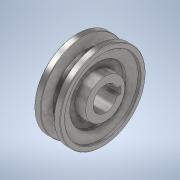
# Autodesk Inventor part: Pulley
Saved by Autodesk Inventor 2021 (Build 250183000, 183)
## iProperties
Created: 2021-07-07
Part Number: Pulley
Material: Steel, Cast
Document SubType Name: Modeling
Designer: MOGIRE
Density: 7.85 g/cm^3
Appearance: Semi-Polished
Author: MOGIRE
Autodesk Inventor part; units mm, degrees
ref_plane "YZ Plane" through (0, 0, 0) normal (1, 0, 0) x (0, 1, 0)
ref_plane "XZ Plane" through (0, 0, 0) normal (0, 1, 0) x (-1, 0, 0)
ref_plane "XY Plane" through (0, 0, 0) normal (0, 0, 1) x (1, 0, 0)
sketch "Sketch1" plane through (0, 0, 0) normal (0, 0, 1) x (1, 0, 0)
  line L0 (0, 0) -> (31.7677, 0)
  line L1 (0, 50) -> (26.4201, 50)
  line L2 (26.4201, 50) -> (55.3898, 50)
  line L3 (55.3898, 50) -> (62.5, 50)
  line L4 (62.5, 50) -> (62.5, 80)
  line L5 (62.5, 80) -> (20, 82.2273)
  line L6 (20, 82.2273) -> (20, 114.4691)
  line L7 (20, 114.4691) -> (32.145, 115.1056)
  line L8 (32.145, 115.1056) -> (42.6931, 154.4717)
  line L9 (42.6931, 154.4717) -> (52.7742, 155)
  line L10 (52.7742, 155) -> (52.7742, 175)
  line L11 (5.5003, 135) -> (16.7702, 135)
  line L12 (16.7702, 135) -> (27.4881, 175)
  line L13 (52.7742, 175) -> (27.4881, 175)
  line L14 (5.5003, 135) -> (0, 135)
  line L15 (0, 50) -> (0, 157.6069) construction
  line L16 (0, 50) -> (-26.4201, 50)
  line L17 (-26.4201, 50) -> (-55.3898, 50)
  line L18 (-55.3898, 50) -> (-62.5, 50)
  line L19 (-62.5, 50) -> (-62.5, 80)
  line L20 (-62.5, 80) -> (-20, 82.2273)
  line L21 (-20, 82.2273) -> (-20, 114.4691)
  line L22 (-20, 114.4691) -> (-32.145, 115.1056)
  line L23 (-32.145, 115.1056) -> (-42.6931, 154.4717)
  line L24 (-42.6931, 154.4717) -> (-52.7742, 155)
  line L25 (-52.7742, 155) -> (-52.7742, 175)
  line L26 (-5.5003, 135) -> (-16.7702, 135)
  line L27 (-16.7702, 135) -> (-27.4881, 175)
  line L28 (-52.7742, 175) -> (-27.4881, 175)
  line L29 (-5.5003, 135) -> (0, 135)
  dimension "d7" = 62.5
  dimension "d8" = 80
  dimension "d9" = 50
  dimension "d14" = 93
  dimension "d16" = 20
  dimension "d20" = 93
  dimension "d21" = 12.145
  dimension "d23" = 108
  dimension "d24" = 93
  dimension "d25" = 155
  dimension "d26" = 175
  dimension "d27" = 20
  constraints: 60 end point, 13 symmetric about line, 4 horizontal, 3 point on line, 3 vertical, 1 coincident, 1 parallel, 1 perpendicular, 1 other
  measures "d7" distance of L3.end L1.start
  measures "d8" vertical distance of point (0, 0) L4.end
  measures "d9" vertical distance of point (0, 0) L3.end
  measures "d14" angle of L5 L6
  measures "d16" distance from line of L6 L1.start
  measures "d20" angle of L6 L7
  measures "d21" horizontal distance of L6.end L7.end
  measures "d23" angle of L7 L8
  measures "d24" angle of L10 L9
  measures "d25" vertical distance of L9.end point (0, 0)
  measures "d26" vertical distance of point (0, 0) L10.end
  measures "d27" distance between parallel lines of L8 L12
revolve "Revolution1" add sketch "Sketch1" angle 360 about axis through (0, 0, 0) along (1, 0, 0)
sketch "Sketch2" plane through (0, 0, 0) normal (1, 0, 0) x (0, 1, 0)
  line L0 (0, 0) -> (-15, 0)
  line L1 (-15, -13.3049) -> (-15, -62.5)
  line L2 (-15, -62.5) -> (15, -62.5)
  line L3 (15, -62.5) -> (15, -13.3049)
  line L4 (15, -13.3049) -> (-15, -13.3049)
  circle A0 centre (0, 0) radius 50 projected
  arc A1 (-15, -47.697) -> (15, -47.697) centre (0, 0) ccw
  dimension "d30" = 15
  dimension "d31" = 62.5
  dimension "d32" = 30
  constraints: 10 end point, 4 point on circle, 3 perpendicular, 2 point on line, 1 centre point, 1 horizontal, 1 vertical
  measures "d30" distance of L0.start L0.end
  measures "d31" distance of L0.end L1.end
  measures "d32" distance of L1.end L2.end
extrude "Extrusion1" cut sketch "Sketch2" against normal mid plane 300 contours L4 L3 A0 L1 | A0 L3 L2 L1 picked at (0, -25.5366)
fillet "Fillet1" radius 2 7 edges at (-27.4881, -175, 0) (27.4881, -175, 0) (52.7742, -175, 0) (52.7742, -155, 0) (-52.7742, -175, 0) (-52.7742, -155, 0) (-32.145, -115.1056, 0)
body "Solid1"
